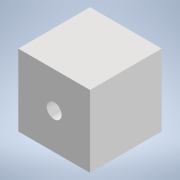
# Autodesk Inventor part: cylinderForCopy
Saved by Autodesk Inventor 2020.2 (Build 242310000, 310)
## iProperties
Created: 2020-01-21
Part Number: cylinderForCopy
Material: Generic
Document SubType Name: Modeling
Designer: robst
Density: 1 g/cm^3
Appearance: Default
Author: robst
Autodesk Inventor part; units mm, degrees
ref_plane "YZ Plane" through (0, 0, 0) normal (1, 0, 0) x (0, 1, 0)
ref_plane "XY Plane" through (0, 0, 0) normal (0, 0, 1) x (1, 0, 0)
sketch "Sketch1" plane through (0, 0, 0) normal (1, 0, 0) x (0, 1, 0)
  line L0 (-25.4, -25.4) -> (-25.4, 25.4)
  line L1 (-25.4, 25.4) -> (25.4, 25.4)
  line L2 (25.4, 25.4) -> (25.4, -25.4)
  line L3 (25.4, -25.4) -> (-25.4, -25.4)
  line L4 (-25.4, -25.4) -> (25.4, 25.4) construction
  line L5 (-25.4, 25.4) -> (25.4, -25.4) construction
  point P0 (0, 0)
  dimension "d0" = 50.8
  dimension "d1" = 50.8
  constraints: 12 end point, 2 midpoint, 2 parallel, 1 perpendicular, 1 vertical
  measures "d0" distance of L0.start L0.end
  measures "d1" distance of L0.end L1.end
extrude "Extrusion1" add sketch "Sketch1" along normal mid plane 50.8
sketch "Sketch2" plane through (-25.4, -25.4, 25.4) normal (0, 0, 1) x (1, 0, 0)
  circle A0 centre (25.4, 25.4) radius 5.2705
  dimension "d4" = 10.541
  constraints: 1 centre point, 1 coincident
  measures "d4" diameter of A0
extrude "Extrusion2" cut sketch "Sketch2" against normal through all
body "Solid1"
